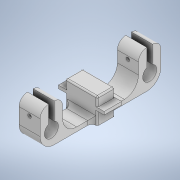
# Autodesk Inventor part: SupportGimbalAdafruit
Saved by Autodesk Inventor 2022 (Build 260153000, 153)
## iProperties
Created: 2021-12-12
Part Number: SupportGimbalAdafruit
Material: Generico
Document SubType Name: Modeling
Designer: narde
Density: 1 g/cm^3
Appearance: Default
Author: narde
Autodesk Inventor part; units mm, degrees
ref_plane "YZ Plane" through (0, 0, 0) normal (1, 0, 0) x (0, 1, 0)
ref_plane "XZ Plane" through (0, 0, 0) normal (0, 1, 0) x (-1, 0, 0)
ref_plane "XY Plane" through (0, 0, 0) normal (0, 0, 1) x (1, 0, 0)
sketch "Schizzo1" plane through (0, 0, 0) normal (0, 1, 0) x (-1, 0, 0)
  line L0 (7.5, 43) -> (-7.5, 43)
  line L1 (-7.5, 43) -> (-7.5, -43)
  line L2 (-7.5, -43) -> (7.5, -43)
  line L3 (7.5, -43) -> (7.5, 43)
  line L4 (7.5, 43) -> (-7.5, -43) construction
  line L5 (-7.5, 43) -> (7.5, -43) construction
  point P0 (0, 0)
  dimension "d0" = 15
  dimension "d1" = 86
  constraints: 12 end point, 2 midpoint, 2 parallel, 1 horizontal, 1 perpendicular
  measures "d0" distance of L2.end L1.end
  measures "d1" distance of L1.end L0.end
extrude "Estrusione1" add sketch "Schizzo1" along normal blind 3
sketch "Schizzo2" plane through (0, 3, 0) normal (0, 1, 0) x (1, 0, 0)
  line L0 (7.5, 43) -> (-7.5, 43)
  line L1 (-7.5, 43) -> (-7.5, 27)
  line L2 (-7.5, 27) -> (7.5, 27)
  line L3 (7.5, 27) -> (7.5, 43)
  line L4 (-7.5, 43) -> (-7.5, -43) projected
  line L5 (7.5, 43) -> (-7.5, 43) projected
  line L6 (-7.5, -43) -> (7.5, -43) projected
  line L7 (7.5, -43) -> (-7.5, -43)
  line L8 (-7.5, -43) -> (-7.5, -27)
  line L9 (-7.5, -27) -> (7.5, -27)
  line L10 (7.5, -27) -> (7.5, -43)
  point P0 (0, 0)
  dimension "d4" = 15
  dimension "d5" = 16
  dimension "d6" = 0
  dimension "d7" = 0
  dimension "d8" = 16
  constraints: 16 end point, 4 parallel, 2 horizontal, 2 perpendicular, 1 point on line
  measures "d4" distance of L2.end L1.end
  measures "d5" distance of L1.end L0.end
  measures "d6" distance between parallel lines of L4 L1
  measures "d7" distance between parallel lines of L5 L0
  measures "d8" distance of L7.end L8.end
extrude "Estrusione2" add sketch "Schizzo2" along normal blind 24
sketch "Schizzo3" plane through (-7.5, 0, -43) normal (-1, 0, 0) x (0, 0, 1)
  line L0 (0, 0) -> (86, 0) projected
  line L1 (0, 0) -> (0, 27) projected
  line L2 (86, 0) -> (86, 27) projected
  circle A0 centre (8, 10) radius 5
  circle A1 centre (78, 10) radius 5
  point P0 (43, 0)
  dimension "d11" = 10
  dimension "d12" = 8
  dimension "d13" = 10
  dimension "d14" = 8
  dimension "d15" = 10
  dimension "d16" = 10
  constraints: 2 centre point, 2 coincident
  measures "d11" distance from line of L0 point (8, 10)
  measures "d12" distance from line of L1 point (8, 10)
  measures "d13" distance from line of L0 point (78, 10)
  measures "d14" distance from line of L2 point (78, 10)
  measures "d15" diameter of A0
  measures "d16" diameter of A1
extrude "Estrusione3" cut sketch "Schizzo3" against normal blind 30
fillet "Raccordo1" radius 10 2 edges at (0, 3, -27) (0, 3, 27)
fillet "Raccordo2" radius 10 2 edges at (0, 0, -43) (0, 0, 43)
sketch "Schizzo4" plane through (0, 27, 0) normal (0, 1, 0) x (1, 0, 0)
  line L0 (7.5, 37) -> (-7.5, 37)
  line L1 (-7.5, 37) -> (-7.5, 33)
  line L2 (-7.5, 33) -> (7.5, 33)
  line L3 (7.5, 33) -> (7.5, 37)
  line L4 (7.5, 27) -> (7.5, 43) projected
  line L5 (7.5, 43) -> (-7.5, 43) projected
  line L6 (7.5, -33) -> (-7.5, -33)
  line L7 (-7.5, -33) -> (-7.5, -37)
  line L8 (-7.5, -37) -> (7.5, -37)
  line L9 (7.5, -37) -> (7.5, -33)
  line L10 (7.5, -43) -> (7.5, -27) projected
  line L11 (-7.5, -43) -> (7.5, -43) projected
  point P0 (0, 0)
  dimension "d21" = 15
  dimension "d22" = 4
  dimension "d23" = 0
  dimension "d24" = 6
  dimension "d25" = 15
  dimension "d26" = 4
  dimension "d27" = 0
  dimension "d28" = 6
  constraints: 16 end point, 4 parallel, 2 horizontal, 2 perpendicular
  measures "d21" distance of L2.end L1.end
  measures "d22" distance of L1.end L0.end
  measures "d23" distance between parallel lines of L4 L3
  measures "d24" distance between parallel lines of L5 L0
  measures "d25" distance of L8.end L7.end
  measures "d26" distance of L7.end L6.end
  measures "d27" distance between parallel lines of L10 L9
  measures "d28" distance between parallel lines of L11 L8
extrude "Estrusione4" cut sketch "Schizzo4" against normal blind 15
sketch "Schizzo5" plane through (7.5, 27, -43) normal (0, 0, -1) x (-1, 0, 0)
  line L0 (0, 0) -> (15, 0) projected
  line L1 (15, -17) -> (15, 0) projected
  circle A0 centre (7.5, -8) radius 1.25
  point P0 (7.5, -27)
  dimension "d31" = 8
  dimension "d32" = 7.5
  dimension "d33" = 2.5
  constraints: 1 centre point, 1 coincident
  measures "d31" distance from line of L0 point (7.5, -8)
  measures "d32" distance from line of L1 point (7.5, -8)
  measures "d33" diameter of A0
extrude "Estrusione5" cut sketch "Schizzo5" against normal blind 86
fillet "Raccordo3" radius 6 4 edges at (0, 27, 43) (0, 27, 27) (0, 27, -27) (0, 27, -43)
sketch "Schizzo6" plane through (0, 0, 0) normal (0, -1, 0) x (1, 0, 0)
  line L0 (-11.4, -6.2) -> (11.4, -6.2)
  line L1 (11.4, -6.2) -> (11.4, 6.2)
  line L2 (11.4, 6.2) -> (-11.4, 6.2)
  line L3 (-11.4, 6.2) -> (-11.4, -6.2)
  line L4 (-11.4, -6.2) -> (11.4, 6.2) construction
  line L5 (11.4, -6.2) -> (-11.4, 6.2) construction
  point P0 (0, 0)
  dimension "d37" = 22.8
  dimension "d38" = 12.4
  constraints: 12 end point, 2 midpoint, 2 parallel, 1 horizontal, 1 perpendicular
  measures "d37" distance of L2.end L1.end
  measures "d38" distance of L1.end L0.end
extrude "Estrusione6" add sketch "Schizzo6" against normal blind 18
sketch "Schizzo7" plane through (11.4, 0, 6.2) normal (1, 0, 0) x (0, 0, -1)
  line L0 (0, 11.5) -> (12.4, 11.5)
  line L1 (12.4, 11.5) -> (12.4, 9.3)
  line L2 (12.4, 9.3) -> (0, 9.3)
  line L3 (0, 9.3) -> (0, 11.5)
  line L4 (0, 11.5) -> (12.4, 9.3) construction
  line L5 (12.4, 11.5) -> (0, 9.3) construction
  line L6 (12.4, 0) -> (0, 0) projected
  line L7 (12.4, 0) -> (12.4, 18) projected
  point P0 (6.2, 0)
  point P1 (6.2, 10.4)
  dimension "d41" = 12.4
  dimension "d42" = 2.2
  dimension "d43" = 9.3
  dimension "d44" = 0
  constraints: 12 end point, 2 midpoint, 2 parallel, 1 horizontal, 1 perpendicular
  measures "d41" distance of L1.end L2.end
  measures "d42" distance of L0.end L1.end
  measures "d43" distance between parallel lines of L6 L2
  measures "d44" distance between parallel lines of L7 L1
extrude "Estrusione7" add sketch "Schizzo7" along normal blind 4.9
sketch "Schizzo8" plane through (-11.4, 0, -6.2) normal (-1, 0, 0) x (0, 0, 1)
  line L0 (0, 11.5) -> (12.4, 11.5)
  line L1 (12.4, 11.5) -> (12.4, 9.3)
  line L2 (12.4, 9.3) -> (0, 9.3)
  line L3 (0, 9.3) -> (0, 11.5)
  line L4 (0, 11.5) -> (12.4, 9.3) construction
  line L5 (12.4, 11.5) -> (0, 9.3) construction
  line L6 (12.4, 0) -> (0, 0) projected
  line L7 (12.4, 0) -> (12.4, 18) projected
  point P0 (6.2, 0)
  point P1 (6.2, 10.4)
  dimension "d47" = 12.4
  dimension "d48" = 2.2
  dimension "d49" = 9.3
  dimension "d50" = 0
  constraints: 12 end point, 2 midpoint, 2 parallel, 1 horizontal, 1 perpendicular
  measures "d47" distance of L1.end L2.end
  measures "d48" distance of L0.end L1.end
  measures "d49" distance between parallel lines of L6 L2
  measures "d50" distance between parallel lines of L7 L1
extrude "Estrusione8" add sketch "Schizzo8" along normal blind 4.9
fillet "Raccordo4" radius 3 2 edges at (0, 3, 6.2) (0, 3, -6.2)
fillet "Raccordo5" radius 1 12 edges at (-11.4, 4.65, 6.2) (-11.4, 14.75, 6.2) (-11.4, 14.75, -6.2) (-11.4, 4.65, -6.2) (-11.4, 18, 0) (0, 18, -6.2) (0, 18, 6.2) (11.4, 4.65, -6.2) (11.4, 14.75, -6.2) (11.4, 18, 0) (11.4, 14.75, 6.2) (11.4, 4.65, 6.2)
fillet "Raccordo6" radius 2.9 8 edges at (-7.5, 4.5, -6.2) (-7.5, 1.5, -6.2) (-7.5, 1.5, 6.2) (-7.5, 4.5, 6.2) (7.5, 4.5, 6.2) (7.5, 1.5, 6.2) (7.5, 1.5, -6.2) (7.5, 4.5, -6.2)
